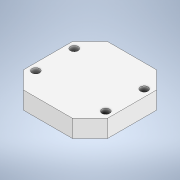
# Autodesk Inventor part: marcor_isolator
Saved by Autodesk Inventor 2020.5 (Build 245400000, 400)
## iProperties
Created: 2019-04-08
Part Number: marcor_isolator
Material: Generic
Document SubType Name: Modeling
Designer: Administrator
Density: 1 g/cm^3
Appearance: Default(1)
Author: Administrator
Autodesk Inventor part; units mm, degrees
ref_plane "YZ Plane" through (0, 0, 0) normal (1, 0, 0) x (0, 1, 0)
ref_plane "XZ Plane" through (0, 0, 0) normal (0, 1, 0) x (-1, 0, 0)
ref_plane "XY Plane" through (0, 0, 0) normal (0, 0, 1) x (1, 0, 0)
sketch "Sketch1" plane through (0, 0, 0) normal (0, 1, 0) x (-1, 0, 0)
  line L0 (10.5005, 23.9999) -> (3.4998, 23.9999)
  line L1 (3.4998, 23.9999) -> (10.5005, 23.9999)
  line L2 (-4.9999, 18.9997) -> (-4.9999, 5.0001)
  line L3 (-0.5002, 23.5006) -> (-4.9999, 18.9997)
  line L4 (-4.9999, 18.9997) -> (-4.9999, 5.0001)
  line L5 (0.0015, 0) -> (13.9982, -0.0002)
  line L6 (-4.9999, 5.0001) -> (0.0015, 0)
  line L7 (0.0015, 0) -> (13.9982, -0.0002)
  line L8 (13.9982, -0.0002) -> (18.9999, 5.0029)
  line L9 (18.9999, 5.0029) -> (19.0001, 19)
  line L10 (18.9999, 5.0029) -> (19.0001, 19)
  line L11 (19.0001, 19) -> (14.4994, 23.4994)
  circle A0 centre (17, 17.4999) radius 0.8
  circle A1 centre (17, 17.4999) radius 0.8
  circle A2 centre (17, 6.5) radius 0.8
  circle A3 centre (17, 6.5) radius 0.8
  circle A4 centre (-3, 17.5) radius 0.8
  circle A5 centre (-3, 17.5) radius 0.8
  circle A6 centre (-3, 6.5) radius 0.8
  circle A7 centre (-3, 17.5) radius 0.8
  line L12 (19.0001, 19) -> (19.0001, 16.4173)
  line L13 (19.0001, 19) -> (19, 15.3998)
  line L14 (19.0001, 19) -> (19, 15.3998)
  line L15 (19.0001, 19) -> (18.3991, 19.6008)
  line L16 (19.0001, 19) -> (18.3998, 19.6001)
  line L17 (19.0001, 19) -> (19, 11.9999)
  line L18 (19, 11.9999) -> (-4.9999, 11.9999)
  line L19 (19, 11.9999) -> (7, 11.9999)
  line L20 (6.9998, -0.0001) -> (7.0002, 23.9999)
  line L21 (-4.8205, 19.6001) -> (-4.8205, 19.6005)
  line L22 (-2.9994, 19.6006) -> (-2.9994, 19.6001)
  line L23 (10.5005, 23.9999) -> (13.9988, 23.9999)
  line L24 (14.4994, 23.4994) -> (13.9988, 23.9999)
  line L25 (3.4998, 23.9999) -> (-0.001, 23.9999)
  line L26 (-0.5002, 23.5006) -> (-0.001, 23.9999)
  point P0 (0, 0)
  point P1 (0, 0)
  point P2 (10, 14.9997)
  point P3 (4.0003, 14.9997)
  point P4 (4.0003, 8.0001)
  point P5 (7, 14.9997)
  point P6 (7, 14.9997)
  point P7 (7, 14.9997)
  point P8 (7, 11.9999)
  point P9 (-4.9999, 15.4002)
  point P10 (-4.9999, 8.6003)
  point P11 (-4.3996, 4.4)
  point P12 (18.3968, 4.3997)
  point P13 (18.9999, 8.6)
  point P14 (19, 15.3998)
  point P15 (18.9999, 8.6)
  dimension "d2" = 1.6
  constraints: 54 end point, 8 centre point, 5 point on line, 4 coincident, 4 collinear, 4 midpoint, 3 horizontal, 3 perpendicular, 1 concentric, 1 parallel
  measures "d2" diameter of A2
extrude "Extrusion1" add sketch "Sketch1" along normal blind 5
hole "Hole1" at (-17, 0, 6.5) at (-17, 0, 17.4999) at (3, 0, 17.5) at (3, 0, 6.5) direction (0, 1, 0) diameter 2.2 end through all clearance for "Countersunk Flat Head Screw ISO 2009/7046" size "M2" standard "ISO"
body "Solid1"
